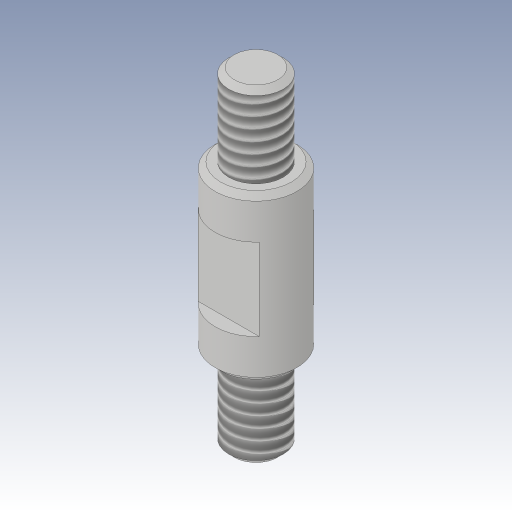
# Autodesk Inventor part: BT006_huenin20_23
Saved by Autodesk Inventor 2023.3 (Build 273359000, 359)
## iProperties
Company: HTBLA Kaindorf
RuleStatus: InUse
Created: 2023-08-29
Part Number: BT006_huenin20_23
Project: Fiberprinter-Hotend
Material: Generisch
Description: Mountingscrew
Document SubType Name: Modeling
Designer: huenin20
Density: 1 g/cm^3
Appearance: Vorgabe
Mass: 0.05602 g
Surface Area: 1.05871 cm^2
Volume: 0.05602 cm^3
AfterDocNew0: iProperties-Editor_aufrufen
Author: nicob
Keywords: 2023
Autodesk Inventor part; units mm, degrees
ref_plane "YZ Plane" through (0, 0, 0) normal (1, 0, 0) x (0, 1, 0)
ref_plane "XZ Plane" through (0, 0, 0) normal (0, 1, 0) x (-1, 0, 0)
ref_plane "XY Plane" through (0, 0, 0) normal (0, 0, 1) x (1, 0, 0)
sketch "Skizze3" plane through (0, 0, 0) normal (1, 0, 0) x (0, 1, 0)
  line L0 (0, 0) -> (0, 12.6925)
  line L1 (0, 0) -> (-1, 0)
  line L2 (-1, 0) -> (-1, 3)
  line L3 (-1, 3) -> (-1.5, 3)
  line L4 (-1.5, 3) -> (-1.5, 9)
  line L5 (-1.5, 9) -> (-1, 9)
  line L6 (-1, 9) -> (-1, 12)
  line L7 (-1, 12) -> (0, 12)
  dimension "d4" = 3
  dimension "d5" = 12
  dimension "d6" = 6
  dimension "d7" = 3
  dimension "d8" = 2
  dimension "d9" = 2
  constraints: 16 end point, 5 perpendicular, 2 vertical, 1 coincident, 1 horizontal, 1 point on line
  measures "d4" diameter of L4 L0
  measures "d5" distance from line of point (0, 0) L7
  measures "d6" distance of L3.end L4.end
  measures "d7" distance between parallel lines of L7 L5
  measures "d8" diameter of L6 L0
  measures "d9" diameter of L2 L0
revolve "Umdrehung1" add sketch "Skizze3" angle 360 about axis through (0, 0, 0) along (0, 0, 1)
chamfer "Fase1" distance 0.2 angle 45 4 edges at (0, 1, 12) (0, 1.5, 9) (0, 1.5, 3) (0, 1, 0)
thread "Gewinde1" size "M2x0.4" class "6g" standard "ISO Metric profile" length 5
thread "Gewinde2" size "M2x0.4" class "6g" standard "ISO Metric profile" length 5
sketch "Skizze4" plane through (0, 0, 0) normal (0, 1, 0) x (-1, 0, 0)
  line L0 (1.5, 3.2) -> (1.5, 8.8) projected
  line L1 (1.5, 4.5) -> (1, 4.5)
  line L2 (1, 4.5) -> (1, 7.5)
  line L3 (1, 7.5) -> (1.5, 7.5)
  line L4 (-0.8, 12) -> (0.8, 12) projected
  line L5 (0, 12) -> (0, 0) construction
  line L6 (-1.5, 4.5) -> (-1, 4.5)
  line L7 (-1, 4.5) -> (-1, 7.5)
  line L8 (-1, 7.5) -> (-1.5, 7.5)
  line L9 (-1.5, 3.2) -> (-1.5, 8.8) projected
  point P0 (1, 6)
  point P1 (1.5, 6)
  dimension "d18" = 3
  dimension "d19" = 0.5
  constraints: 14 end point, 4 symmetric about line, 3 midpoint, 2 perpendicular, 2 point on line, 1 horizontal, 1 horizontal alignment, 1 vertical
  measures "d18" distance of L1.end L2.end
  measures "d19" distance between parallel lines of L0 L2
extrude "Extrusion3" cut sketch "Skizze4" along normal through all both and the other way through all
equation "\"d9\" = d8"
